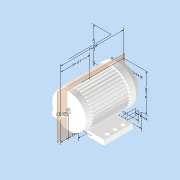
# Autodesk Inventor part: 43010400
Saved by Autodesk Inventor 2021 (Build 250183000, 183)
## iProperties
Category: PARTsolutions
Company: MAEDLER
Created: 2024-03-16
Part Number: 43010400
Material: Generic
Catalog Web Link: www.cadenas.de
Description: MAE-DNM-SM/I-B3-6/POLIG-Standard Three-Phase Motors SM/I, Model B3, 6-polig, approx. 1000 1/min.
Vendor: MAEDLER
Document SubType Name: Modeling
Designer: psAdmin
Manufacturer: MAEDLER
Mass: 6500 g
Surface Area: 2023.36 cm^2
Volume: 3410.98 cm^3
Density: 1 g/cm^3
Appearance: PSOLRGB-235-235-235
PSOL_IDENT_0: {$CADENAS_DATA/23d-libs/maedler/getriebe_u_getriebemotoren/drehstrom_normmotoren/d-nm_sm1_6pol_b3.pr
PSOL_IDENT_1: j},173 {VTYP=3D},{NB=43010400},{LINA=43010400},{NN=MAE-DNM-SM/I-B3-6/POLIG},{DATE=09.12.2023 00:31:4
PSOL_IDENT_2: 6},{GEOMDATE=01.12.2023 07:27:40},{VERSION=},{LINEID=20},{WBVAR=},{WBNUMERIC=}  {NB=43010400},{LINA=
PSOL_IDENT_3: 43010400},{KT=DUMMY},{ARTNR=43010400},{WEBSHOP=Produktdetails / Katalogseite / Montageanleitung},{MA
PSOL_IDENT_4: TK=Aluminium},{MAT=Rippengehäuse: Alu-Druckguss, Lagerschilder: Druckguss, Radiallüfter: Kunststoff,
PSOL_IDENT_5: Lüfterhaube: Stahlblech},{PDN=6-polig / ca. 1000 1/min.},{BG=71},{BF=B3},{IE=IE2},{LE=0.25},{DZ=900
PSOL_IDENT_6: },{J=0.0013},{LAN=59 / - / -},{STR=0.87},{LF=0.70},{NM=2.65},{ADM=2.1},{AS=4.0},{MDM=2.2},{GEW=6.5},
PSOL_IDENT_7: {CTN=85015100},{A=112},{B=90},{C=45},{D=14 j6},{E=30},{F=238},{G=185},{H=71},{K=7},{I=108},{L=137},{
PSOL_IDENT_8: P=24},{R=144},{S=10},{C1=85.5},{F1=280},{G1=125},{X=111},{Y=20},{W=88},{BK=5},{TK=16.0},{PGV=Pg11},{
PSOL_IDENT_9: GWB=M5 x 0.8},{DD=14},{FK=9.5},{XTK1=2.3},{GB1=5},{GB2=0.80},{Z=1},{KB=94},{KL=94},{IB=9.0},{KK=18.6
PSOL_IDENT_10: },{AL=24},{SW=22},{DIST=6.850}
NB: 43010400
NN: MAE-DNM-SM/I-B3-6/POLIG
NT: Standard Three-Phase Motors SM/I, Model B3, 6-polig, approx. 1000 1/min.
NBSYN: $ARTNR.
LINA: 43010400
CATALOG: Mädler
ARTNR: 43010400
WEBSHOP: https://maedler.de/ShopSearch?query=43010400
MATK: Aluminium
MAT: Finned housing: die-cast aluminium, end shields: Die-cast, radial fan: Plastic, fan cover: Sheet steel
PDN: 6 Poles / approx. 1000 1/min.
BG: 71
BF: B3
IE: IE2
LE: 0.25
DZ: 900
J: 0.0013
LAN: 59 / - / -
STR: 0.87
LF: 0.7
NM: 2.65
ADM: 2.1
AS: 4
MDM: 2.2
GEW: 6.5
CTN: 85015100
A: 112
B: 90
C: 45
D: 14 j6
E: 30
F: 238
G: 185
H: 71
K: 7
I: 108
L: 137
P: 24
R: 144
S: 10
G1: 125
X: 111
W: 88
BK: 5
TK: 16
PGV: Pg11
GWB: M5 x 0.8
SUPPLIER: MAEDLER
ARTICLENO: 43010400
BOMINFO: 43010400
CREATOR: CADENAS GmbH
Title: 43010400
Author: Cadenas PARTsolutions
Comments: Standard Three-Phase Motors SM/I, Model B3, 6-polig, approx. 1000 1/min.
Autodesk Inventor part; units mm, degrees
ref_plane "XZ Plane" through (0, 0, 0) normal (0, 1, 0) x (-1, 0, 0)
ref_plane "XY Plane" through (0, 0, 0) normal (0, 0, 1) x (1, 0, 0)
sketch "Skizze_3" plane through (0, 0, 0) normal (1, 0, 0) x (0, 1, 0)
  line L0 (0, 184) -> (0, 232)
  line L1 (7, 208) -> (10.5, 208)
  line L2 (10.5, 208) -> (10.5, 206)
  line L3 (10.5, 206) -> (63.9, 206)
  line L4 (63.9, 206) -> (63.9, 184)
  line L5 (63.9, 184) -> (0, 184)
  line L6 (0, 184) -> (0, 232)
  line L7 (7, 208) -> (7, 232)
  line L8 (7, 232) -> (0, 232)
  dimension "d64" = 2
  dimension "d65" = 3.5
  dimension "d68" = 53.4
  dimension "d69" = 22
  dimension "d70" = 63.9
  dimension "d71" = 24
  constraints: 18 end point, 1 perpendicular, 1 vertical
  measures "d64" distance of L1.end L2.end
  measures "d65" distance of L1.start L1.end
  measures "d68" distance of L2.end L3.end
  measures "d69" distance of L3.end L4.end
  measures "d70" distance of L4.end L5.end
  measures "d71" distance of L1.start L7.end
revolve "Revolution1" add sketch "Skizze_3" angle 360 about axis through (0, 0, 184) along (0, 0, -1)
sketch "Sketch_1" plane through (0, 0, 184) normal (0, 0, 1) x (1, 0, 0)
  arc A0 (-70.0009, 1.0346) -> (-70.0009, -1.0346) centre (-69.9647, 0) ccw
  line L0 (-70.0009, -1.0346) -> (-65.7533, -1.183)
  arc A1 (-63.8255, -3.0852) -> (-65.7533, -1.183) centre (-65.8231, -3.1818) ccw
  arc A2 (-63.8255, -3.0852) -> (-63.703, -5.0135) centre (0, 0) ccw
  arc A3 (-63.703, -5.0135) -> (-63.5223, -6.9373) centre (0, 0) ccw
  arc A4 (-65.1289, -9.1177) -> (-63.5223, -6.9373) centre (-65.5105, -7.1544) ccw
  line L1 (-65.1289, -9.1177) -> (-69.3009, -9.9286)
  arc A5 (-69.3009, -9.9286) -> (-68.9772, -11.9725) centre (-69.1033, -10.9449) ccw
  line L2 (-68.9772, -11.9725) -> (-64.7588, -11.4545)
  arc A6 (-62.5571, -13.0317) -> (-64.7588, -11.4545) centre (-64.515, -13.4396) ccw
  arc A7 (-62.5571, -13.0317) -> (-62.1344, -14.9172) centre (0, 0) ccw
  arc A8 (-62.1344, -14.9172) -> (-61.655, -16.789) centre (0, 0) ccw
  arc A9 (-62.9007, -19.1938) -> (-61.655, -16.789) centre (-63.5847, -17.3144) ccw
  line L3 (-62.9007, -19.1938) -> (-66.8945, -20.6474)
  arc A10 (-66.8945, -20.6474) -> (-66.255, -22.6155) centre (-66.5404, -21.6203) ccw
  line L4 (-66.255, -22.6155) -> (-62.1696, -21.444)
  arc A11 (-59.7483, -22.6573) -> (-62.1696, -21.444) centre (-61.6183, -23.3665) ccw
  arc A12 (-59.7483, -22.6573) -> (-59.0359, -24.4535) centre (0, 0) ccw
  arc A13 (-59.0359, -24.4535) -> (-58.2696, -26.2272) centre (0, 0) ccw
  arc A14 (-59.1237, -28.7974) -> (-58.2696, -26.2272) centre (-60.0933, -27.0481) ccw
  line L5 (-59.1237, -28.7974) -> (-62.8409, -30.8578)
  arc A15 (-62.8409, -30.8578) -> (-61.9015, -32.7016) centre (-62.339, -31.7633) ccw
  line L6 (-61.9015, -32.7016) -> (-58.0496, -30.9054)
  arc A16 (-55.4683, -31.7251) -> (-58.0496, -30.9054) centre (-57.2044, -32.718) ccw
  arc A17 (-55.4683, -31.7251) -> (-54.4837, -33.3877) centre (0, 0) ccw
  arc A18 (-54.4837, -33.3877) -> (-53.4493, -35.0197) centre (0, 0) ccw
  arc A19 (-53.8909, -37.6918) -> (-53.4493, -35.0197) centre (-55.1222, -36.1158) ccw
  line L7 (-53.8909, -37.6918) -> (-57.24, -40.3084)
  arc A20 (-57.24, -40.3084) -> (-56.0237, -41.9825) centre (-56.6027, -41.1242) ccw
  line L8 (-56.0237, -41.9825) -> (-52.5002, -39.6059)
  arc A21 (-49.8225, -40.0116) -> (-52.5002, -39.6059) centre (-51.3819, -41.264) ccw
  arc A22 (-49.8225, -40.0116) -> (-48.5899, -41.4997) centre (0, 0) ccw
  arc A23 (-48.5899, -41.4997) -> (-47.313, -42.9499) centre (0, 0) ccw
  arc A24 (-47.3311, -45.6582) -> (-47.313, -42.9499) centre (-48.7938, -44.2942) ccw
  line L9 (-47.3311, -45.6582) -> (-50.2297, -48.7665)
  arc A25 (-50.2297, -48.7665) -> (-48.7665, -50.2297) centre (-49.4725, -49.4725) ccw
  line L10 (-48.7665, -50.2297) -> (-45.6582, -47.3311)
  arc A26 (-42.9499, -47.313) -> (-45.6582, -47.3311) centre (-44.2942, -48.7938) ccw
  arc A27 (-42.9499, -47.313) -> (-41.4997, -48.5899) centre (0, 0) ccw
  arc A28 (-41.4997, -48.5899) -> (-40.0116, -49.8225) centre (0, 0) ccw
  arc A29 (-39.6059, -52.5002) -> (-40.0116, -49.8225) centre (-41.264, -51.3819) ccw
  line L11 (-39.6059, -52.5002) -> (-41.9825, -56.0237)
  arc A30 (-41.9825, -56.0237) -> (-40.3084, -57.24) centre (-41.1242, -56.6027) ccw
  line L12 (-40.3084, -57.24) -> (-37.6918, -53.8909)
  arc A31 (-35.0197, -53.4493) -> (-37.6918, -53.8909) centre (-36.1158, -55.1222) ccw
  arc A32 (-35.0197, -53.4493) -> (-33.3877, -54.4837) centre (0, 0) ccw
  arc A33 (-33.3877, -54.4837) -> (-31.7251, -55.4683) centre (0, 0) ccw
  arc A34 (-30.9054, -58.0496) -> (-31.7251, -55.4683) centre (-32.718, -57.2044) ccw
  line L13 (-30.9054, -58.0496) -> (-32.7016, -61.9015)
  arc A35 (-32.7016, -61.9015) -> (-30.8578, -62.8409) centre (-31.7633, -62.339) ccw
  line L14 (-30.8578, -62.8409) -> (-28.7974, -59.1237)
  arc A36 (-26.2272, -58.2696) -> (-28.7974, -59.1237) centre (-27.0481, -60.0933) ccw
  arc A37 (-26.2272, -58.2696) -> (-24.4535, -59.0359) centre (0, 0) ccw
  arc A38 (-24.4535, -59.0359) -> (-22.6573, -59.7483) centre (0, 0) ccw
  arc A39 (-21.444, -62.1696) -> (-22.6573, -59.7483) centre (-23.3665, -61.6183) ccw
  line L15 (-21.444, -62.1696) -> (-22.6155, -66.255)
  arc A40 (-22.6155, -66.255) -> (-20.6474, -66.8945) centre (-21.6203, -66.5404) ccw
  line L16 (-20.6474, -66.8945) -> (-19.1938, -62.9007)
  arc A41 (-16.789, -61.655) -> (-19.1938, -62.9007) centre (-17.3144, -63.5847) ccw
  arc A42 (-16.789, -61.655) -> (-14.9172, -62.1344) centre (0, 0) ccw
  arc A43 (-14.9172, -62.1344) -> (-13.0317, -62.5571) centre (0, 0) ccw
  arc A44 (-11.4545, -64.7588) -> (-13.0317, -62.5571) centre (-13.4396, -64.515) ccw
  line L17 (-11.4545, -64.7588) -> (-11.9725, -68.9772)
  arc A45 (-11.9725, -68.9772) -> (-9.9286, -69.3009) centre (-10.9449, -69.1033) ccw
  line L18 (-9.9286, -69.3009) -> (-9.1177, -65.1289)
  arc A46 (-6.9373, -63.5223) -> (-9.1177, -65.1289) centre (-7.1544, -65.5105) ccw
  arc A47 (-6.9373, -63.5223) -> (-5.0135, -63.703) centre (0, 0) ccw
  arc A48 (-5.0135, -63.703) -> (-3.0852, -63.8255) centre (0, 0) ccw
  arc A49 (-1.183, -65.7533) -> (-3.0852, -63.8255) centre (-3.1818, -65.8231) ccw
  line L19 (-1.183, -65.7533) -> (-1.0346, -70.0009)
  arc A50 (-1.0346, -70.0009) -> (1.0346, -70.0009) centre (0, -69.9647) ccw
  line L20 (1.0346, -70.0009) -> (1.183, -65.7533)
  arc A51 (3.0852, -63.8255) -> (1.183, -65.7533) centre (3.1818, -65.8231) ccw
  arc A52 (3.0852, -63.8255) -> (5.0135, -63.703) centre (0, 0) ccw
  arc A53 (5.0135, -63.703) -> (6.9373, -63.5223) centre (0, 0) ccw
  arc A54 (9.1177, -65.1289) -> (6.9373, -63.5223) centre (7.1544, -65.5105) ccw
  line L21 (9.1177, -65.1289) -> (9.9286, -69.3009)
  arc A55 (9.9286, -69.3009) -> (11.9725, -68.9772) centre (10.9449, -69.1033) ccw
  line L22 (11.9725, -68.9772) -> (11.4545, -64.7588)
  arc A56 (13.0317, -62.5571) -> (11.4545, -64.7588) centre (13.4396, -64.515) ccw
  arc A57 (13.0317, -62.5571) -> (14.9172, -62.1344) centre (0, 0) ccw
  arc A58 (14.9172, -62.1344) -> (16.789, -61.655) centre (0, 0) ccw
  arc A59 (19.1938, -62.9007) -> (16.789, -61.655) centre (17.3144, -63.5847) ccw
  line L23 (19.1938, -62.9007) -> (20.6474, -66.8945)
  arc A60 (20.6474, -66.8945) -> (22.6155, -66.255) centre (21.6203, -66.5404) ccw
  line L24 (22.6155, -66.255) -> (21.444, -62.1696)
  arc A61 (22.6573, -59.7483) -> (21.444, -62.1696) centre (23.3665, -61.6183) ccw
  arc A62 (22.6573, -59.7483) -> (24.4535, -59.0359) centre (0, 0) ccw
  arc A63 (24.4535, -59.0359) -> (26.2272, -58.2696) centre (0, 0) ccw
  arc A64 (28.7974, -59.1237) -> (26.2272, -58.2696) centre (27.0481, -60.0933) ccw
  line L25 (28.7974, -59.1237) -> (30.8578, -62.8409)
  arc A65 (30.8578, -62.8409) -> (32.7016, -61.9015) centre (31.7633, -62.339) ccw
  line L26 (32.7016, -61.9015) -> (30.9054, -58.0496)
  arc A66 (31.7251, -55.4683) -> (30.9054, -58.0496) centre (32.718, -57.2044) ccw
  arc A67 (31.7251, -55.4683) -> (33.3877, -54.4837) centre (0, 0) ccw
  arc A68 (33.3877, -54.4837) -> (35.0197, -53.4493) centre (0, 0) ccw
  arc A69 (37.6918, -53.8909) -> (35.0197, -53.4493) centre (36.1158, -55.1222) ccw
  line L27 (37.6918, -53.8909) -> (40.3084, -57.24)
  arc A70 (40.3084, -57.24) -> (41.9825, -56.0237) centre (41.1242, -56.6027) ccw
  line L28 (41.9825, -56.0237) -> (39.6059, -52.5002)
  arc A71 (40.0116, -49.8225) -> (39.6059, -52.5002) centre (41.264, -51.3819) ccw
  arc A72 (40.0116, -49.8225) -> (41.4997, -48.5899) centre (0, 0) ccw
  arc A73 (41.4997, -48.5899) -> (42.9499, -47.313) centre (0, 0) ccw
  arc A74 (45.6582, -47.3311) -> (42.9499, -47.313) centre (44.2942, -48.7938) ccw
  line L29 (45.6582, -47.3311) -> (48.7665, -50.2297)
  arc A75 (48.7665, -50.2297) -> (50.2297, -48.7665) centre (49.4725, -49.4725) ccw
  line L30 (50.2297, -48.7665) -> (47.3311, -45.6582)
  arc A76 (47.313, -42.9499) -> (47.3311, -45.6582) centre (48.7938, -44.2942) ccw
  arc A77 (47.313, -42.9499) -> (48.5899, -41.4997) centre (0, 0) ccw
  arc A78 (48.5899, -41.4997) -> (49.8225, -40.0116) centre (0, 0) ccw
  arc A79 (52.5002, -39.6059) -> (49.8225, -40.0116) centre (51.3819, -41.264) ccw
  line L31 (52.5002, -39.6059) -> (56.0237, -41.9825)
  arc A80 (56.0237, -41.9825) -> (57.24, -40.3084) centre (56.6027, -41.1242) ccw
  line L32 (57.24, -40.3084) -> (53.8909, -37.6918)
  arc A81 (53.4493, -35.0197) -> (53.8909, -37.6918) centre (55.1222, -36.1158) ccw
  arc A82 (53.4493, -35.0197) -> (54.4837, -33.3877) centre (0, 0) ccw
  arc A83 (54.4837, -33.3877) -> (55.4683, -31.7251) centre (0, 0) ccw
  arc A84 (58.0496, -30.9054) -> (55.4683, -31.7251) centre (57.2044, -32.718) ccw
  line L33 (58.0496, -30.9054) -> (61.9015, -32.7016)
  arc A85 (61.9015, -32.7016) -> (62.8409, -30.8578) centre (62.339, -31.7633) ccw
  line L34 (62.8409, -30.8578) -> (59.1237, -28.7974)
  arc A86 (58.2696, -26.2272) -> (59.1237, -28.7974) centre (60.0933, -27.0481) ccw
  arc A87 (58.2696, -26.2272) -> (59.0359, -24.4535) centre (0, 0) ccw
  arc A88 (59.0359, -24.4535) -> (59.7483, -22.6573) centre (0, 0) ccw
  arc A89 (62.1696, -21.444) -> (59.7483, -22.6573) centre (61.6183, -23.3665) ccw
  line L35 (62.1696, -21.444) -> (66.255, -22.6155)
  arc A90 (66.255, -22.6155) -> (66.8945, -20.6474) centre (66.5404, -21.6203) ccw
  line L36 (66.8945, -20.6474) -> (62.9007, -19.1938)
  arc A91 (61.655, -16.789) -> (62.9007, -19.1938) centre (63.5847, -17.3144) ccw
  arc A92 (61.655, -16.789) -> (62.1344, -14.9172) centre (0, 0) ccw
  arc A93 (62.1344, -14.9172) -> (62.5571, -13.0317) centre (0, 0) ccw
  arc A94 (64.7588, -11.4545) -> (62.5571, -13.0317) centre (64.515, -13.4396) ccw
  line L37 (64.7588, -11.4545) -> (68.9772, -11.9725)
  arc A95 (68.9772, -11.9725) -> (69.3009, -9.9286) centre (69.1033, -10.9449) ccw
  line L38 (69.3009, -9.9286) -> (65.1289, -9.1177)
  arc A96 (63.5223, -6.9373) -> (65.1289, -9.1177) centre (65.5105, -7.1544) ccw
  arc A97 (63.5223, -6.9373) -> (63.703, -5.0135) centre (0, 0) ccw
  arc A98 (63.703, -5.0135) -> (63.8255, -3.0852) centre (0, 0) ccw
  arc A99 (65.7533, -1.183) -> (63.8255, -3.0852) centre (65.8231, -3.1818) ccw
  line L39 (65.7533, -1.183) -> (70.0009, -1.0346)
  arc A100 (70.0009, -1.0346) -> (70.0009, 1.0346) centre (69.9647, 0) ccw
  line L40 (70.0009, 1.0346) -> (65.7533, 1.183)
  arc A101 (63.8255, 3.0852) -> (65.7533, 1.183) centre (65.8231, 3.1818) ccw
  arc A102 (63.8255, 3.0852) -> (63.703, 5.0135) centre (0, 0) ccw
  arc A103 (63.703, 5.0135) -> (63.5223, 6.9373) centre (0, 0) ccw
  arc A104 (65.1289, 9.1177) -> (63.5223, 6.9373) centre (65.5105, 7.1544) ccw
  line L41 (65.1289, 9.1177) -> (69.3009, 9.9286)
  arc A105 (69.3009, 9.9286) -> (68.9772, 11.9725) centre (69.1033, 10.9449) ccw
  line L42 (68.9772, 11.9725) -> (64.7588, 11.4545)
  arc A106 (62.5571, 13.0317) -> (64.7588, 11.4545) centre (64.515, 13.4396) ccw
  arc A107 (62.5571, 13.0317) -> (62.1344, 14.9172) centre (0, 0) ccw
  arc A108 (62.1344, 14.9172) -> (61.655, 16.789) centre (0, 0) ccw
  arc A109 (62.9007, 19.1938) -> (61.655, 16.789) centre (63.5847, 17.3144) ccw
  line L43 (62.9007, 19.1938) -> (66.8945, 20.6474)
  arc A110 (66.8945, 20.6474) -> (66.255, 22.6155) centre (66.5404, 21.6203) ccw
  line L44 (66.255, 22.6155) -> (62.1696, 21.444)
  arc A111 (59.7483, 22.6573) -> (62.1696, 21.444) centre (61.6183, 23.3665) ccw
  arc A112 (59.7483, 22.6573) -> (59.0359, 24.4535) centre (0, 0) ccw
  arc A113 (59.0359, 24.4535) -> (58.2696, 26.2272) centre (0, 0) ccw
  arc A114 (59.1237, 28.7974) -> (58.2696, 26.2272) centre (60.0933, 27.0481) ccw
  line L45 (59.1237, 28.7974) -> (62.8409, 30.8578)
  arc A115 (62.8409, 30.8578) -> (61.9015, 32.7016) centre (62.339, 31.7633) ccw
  line L46 (61.9015, 32.7016) -> (58.0496, 30.9054)
  arc A116 (55.4683, 31.7251) -> (58.0496, 30.9054) centre (57.2044, 32.718) ccw
  arc A117 (55.4683, 31.7251) -> (54.4837, 33.3877) centre (0, 0) ccw
  arc A118 (54.4837, 33.3877) -> (53.4493, 35.0197) centre (0, 0) ccw
  arc A119 (53.8909, 37.6918) -> (53.4493, 35.0197) centre (55.1222, 36.1158) ccw
  line L47 (53.8909, 37.6918) -> (57.24, 40.3084)
  arc A120 (57.24, 40.3084) -> (56.0237, 41.9825) centre (56.6027, 41.1242) ccw
  line L48 (56.0237, 41.9825) -> (52.5002, 39.6059)
  arc A121 (49.8225, 40.0116) -> (52.5002, 39.6059) centre (51.3819, 41.264) ccw
  arc A122 (49.8225, 40.0116) -> (48.5899, 41.4997) centre (0, 0) ccw
  arc A123 (48.5899, 41.4997) -> (47.313, 42.9499) centre (0, 0) ccw
  arc A124 (47.3311, 45.6582) -> (47.313, 42.9499) centre (48.7938, 44.2942) ccw
  line L49 (47.3311, 45.6582) -> (50.2297, 48.7665)
  arc A125 (50.2297, 48.7665) -> (48.7665, 50.2297) centre (49.4725, 49.4725) ccw
  line L50 (48.7665, 50.2297) -> (45.6582, 47.3311)
  arc A126 (42.9499, 47.313) -> (45.6582, 47.3311) centre (44.2942, 48.7938) ccw
  arc A127 (42.9499, 47.313) -> (41.4997, 48.5899) centre (0, 0) ccw
  arc A128 (41.4997, 48.5899) -> (40.0116, 49.8225) centre (0, 0) ccw
  arc A129 (39.6059, 52.5002) -> (40.0116, 49.8225) centre (41.264, 51.3819) ccw
  line L51 (39.6059, 52.5002) -> (41.9825, 56.0237)
  arc A130 (41.9825, 56.0237) -> (40.3084, 57.24) centre (41.1242, 56.6027) ccw
  line L52 (40.3084, 57.24) -> (37.6918, 53.8909)
  arc A131 (35.0197, 53.4493) -> (37.6918, 53.8909) centre (36.1158, 55.1222) ccw
  arc A132 (35.0197, 53.4493) -> (33.3877, 54.4837) centre (0, 0) ccw
  arc A133 (33.3877, 54.4837) -> (31.7251, 55.4683) centre (0, 0) ccw
  arc A134 (30.9054, 58.0496) -> (31.7251, 55.4683) centre (32.718, 57.2044) ccw
  line L53 (30.9054, 58.0496) -> (32.7016, 61.9015)
  arc A135 (32.7016, 61.9015) -> (30.8578, 62.8409) centre (31.7633, 62.339) ccw
  line L54 (30.8578, 62.8409) -> (28.7974, 59.1237)
  arc A136 (26.2272, 58.2696) -> (28.7974, 59.1237) centre (27.0481, 60.0933) ccw
  arc A137 (26.2272, 58.2696) -> (24.4535, 59.0359) centre (0, 0) ccw
  arc A138 (24.4535, 59.0359) -> (22.6573, 59.7483) centre (0, 0) ccw
  arc A139 (21.444, 62.1696) -> (22.6573, 59.7483) centre (23.3665, 61.6183) ccw
  line L55 (21.444, 62.1696) -> (22.6155, 66.255)
  arc A140 (22.6155, 66.255) -> (20.6474, 66.8945) centre (21.6203, 66.5404) ccw
  line L56 (20.6474, 66.8945) -> (19.1938, 62.9007)
  arc A141 (16.789, 61.655) -> (19.1938, 62.9007) centre (17.3144, 63.5847) ccw
  arc A142 (16.789, 61.655) -> (14.9172, 62.1344) centre (0, 0) ccw
  arc A143 (14.9172, 62.1344) -> (13.0317, 62.5571) centre (0, 0) ccw
  arc A144 (11.4545, 64.7588) -> (13.0317, 62.5571) centre (13.4396, 64.515) ccw
  line L57 (11.4545, 64.7588) -> (11.9725, 68.9772)
  arc A145 (11.9725, 68.9772) -> (9.9286, 69.3009) centre (10.9449, 69.1033) ccw
  line L58 (9.9286, 69.3009) -> (9.1177, 65.1289)
  arc A146 (6.9373, 63.5223) -> (9.1177, 65.1289) centre (7.1544, 65.5105) ccw
  arc A147 (6.9373, 63.5223) -> (5.0135, 63.703) centre (0, 0) ccw
  arc A148 (5.0135, 63.703) -> (3.0852, 63.8255) centre (0, 0) ccw
  arc A149 (1.183, 65.7533) -> (3.0852, 63.8255) centre (3.1818, 65.8231) ccw
  line L59 (1.183, 65.7533) -> (1.0346, 70.0009)
  arc A150 (1.0346, 70.0009) -> (-1.0346, 70.0009) centre (0, 69.9647) ccw
  line L60 (-1.0346, 70.0009) -> (-1.183, 65.7533)
  arc A151 (-3.0852, 63.8255) -> (-1.183, 65.7533) centre (-3.1818, 65.8231) ccw
  arc A152 (-3.0852, 63.8255) -> (-5.0135, 63.703) centre (0, 0) ccw
  arc A153 (-5.0135, 63.703) -> (-6.9373, 63.5223) centre (0, 0) ccw
  arc A154 (-9.1177, 65.1289) -> (-6.9373, 63.5223) centre (-7.1544, 65.5105) ccw
  line L61 (-9.1177, 65.1289) -> (-9.9286, 69.3009)
  arc A155 (-9.9286, 69.3009) -> (-11.9725, 68.9772) centre (-10.9449, 69.1033) ccw
  line L62 (-11.9725, 68.9772) -> (-11.4545, 64.7588)
  arc A156 (-13.0317, 62.5571) -> (-11.4545, 64.7588) centre (-13.4396, 64.515) ccw
  arc A157 (-13.0317, 62.5571) -> (-14.9172, 62.1344) centre (0, 0) ccw
  arc A158 (-14.9172, 62.1344) -> (-16.789, 61.655) centre (0, 0) ccw
  arc A159 (-19.1938, 62.9007) -> (-16.789, 61.655) centre (-17.3144, 63.5847) ccw
  line L63 (-19.1938, 62.9007) -> (-20.6474, 66.8945)
  arc A160 (-20.6474, 66.8945) -> (-22.6155, 66.255) centre (-21.6203, 66.5404) ccw
  line L64 (-22.6155, 66.255) -> (-21.444, 62.1696)
  arc A161 (-22.6573, 59.7483) -> (-21.444, 62.1696) centre (-23.3665, 61.6183) ccw
  arc A162 (-22.6573, 59.7483) -> (-24.4535, 59.0359) centre (0, 0) ccw
  arc A163 (-24.4535, 59.0359) -> (-26.2272, 58.2696) centre (0, 0) ccw
  arc A164 (-28.7974, 59.1237) -> (-26.2272, 58.2696) centre (-27.0481, 60.0933) ccw
  line L65 (-28.7974, 59.1237) -> (-30.8578, 62.8409)
  arc A165 (-30.8578, 62.8409) -> (-32.7016, 61.9015) centre (-31.7633, 62.339) ccw
  line L66 (-32.7016, 61.9015) -> (-30.9054, 58.0496)
  arc A166 (-31.7251, 55.4683) -> (-30.9054, 58.0496) centre (-32.718, 57.2044) ccw
  arc A167 (-31.7251, 55.4683) -> (-33.3877, 54.4837) centre (0, 0) ccw
  arc A168 (-33.3877, 54.4837) -> (-35.0197, 53.4493) centre (0, 0) ccw
  arc A169 (-37.6918, 53.8909) -> (-35.0197, 53.4493) centre (-36.1158, 55.1222) ccw
  line L67 (-37.6918, 53.8909) -> (-40.3084, 57.24)
  arc A170 (-40.3084, 57.24) -> (-41.9825, 56.0237) centre (-41.1242, 56.6027) ccw
  line L68 (-41.9825, 56.0237) -> (-39.6059, 52.5002)
  arc A171 (-40.0116, 49.8225) -> (-39.6059, 52.5002) centre (-41.264, 51.3819) ccw
  arc A172 (-40.0116, 49.8225) -> (-41.4997, 48.5899) centre (0, 0) ccw
  arc A173 (-41.4997, 48.5899) -> (-42.9499, 47.313) centre (0, 0) ccw
  arc A174 (-45.6582, 47.3311) -> (-42.9499, 47.313) centre (-44.2942, 48.7938) ccw
  line L69 (-45.6582, 47.3311) -> (-48.7665, 50.2297)
  arc A175 (-48.7665, 50.2297) -> (-50.2297, 48.7665) centre (-49.4725, 49.4725) ccw
  line L70 (-50.2297, 48.7665) -> (-47.3311, 45.6582)
  arc A176 (-47.313, 42.9499) -> (-47.3311, 45.6582) centre (-48.7938, 44.2942) ccw
  arc A177 (-47.313, 42.9499) -> (-48.5899, 41.4997) centre (0, 0) ccw
  arc A178 (-48.5899, 41.4997) -> (-49.8225, 40.0116) centre (0, 0) ccw
  arc A179 (-52.5002, 39.6059) -> (-49.8225, 40.0116) centre (-51.3819, 41.264) ccw
  line L71 (-52.5002, 39.6059) -> (-56.0237, 41.9825)
  arc A180 (-56.0237, 41.9825) -> (-57.24, 40.3084) centre (-56.6027, 41.1242) ccw
  line L72 (-57.24, 40.3084) -> (-53.8909, 37.6918)
  arc A181 (-53.4493, 35.0197) -> (-53.8909, 37.6918) centre (-55.1222, 36.1158) ccw
  arc A182 (-53.4493, 35.0197) -> (-54.4837, 33.3877) centre (0, 0) ccw
  arc A183 (-54.4837, 33.3877) -> (-55.4683, 31.7251) centre (0, 0) ccw
  arc A184 (-58.0496, 30.9054) -> (-55.4683, 31.7251) centre (-57.2044, 32.718) ccw
  line L73 (-58.0496, 30.9054) -> (-61.9015, 32.7016)
  arc A185 (-61.9015, 32.7016) -> (-62.8409, 30.8578) centre (-62.339, 31.7633) ccw
  line L74 (-62.8409, 30.8578) -> (-59.1237, 28.7974)
  arc A186 (-58.2696, 26.2272) -> (-59.1237, 28.7974) centre (-60.0933, 27.0481) ccw
  arc A187 (-58.2696, 26.2272) -> (-59.0359, 24.4535) centre (0, 0) ccw
  arc A188 (-59.0359, 24.4535) -> (-59.7483, 22.6573) centre (0, 0) ccw
  arc A189 (-62.1696, 21.444) -> (-59.7483, 22.6573) centre (-61.6183, 23.3665) ccw
  line L75 (-62.1696, 21.444) -> (-66.255, 22.6155)
  arc A190 (-66.255, 22.6155) -> (-66.8945, 20.6474) centre (-66.5404, 21.6203) ccw
  line L76 (-66.8945, 20.6474) -> (-62.9007, 19.1938)
  arc A191 (-61.655, 16.789) -> (-62.9007, 19.1938) centre (-63.5847, 17.3144) ccw
  arc A192 (-61.655, 16.789) -> (-62.1344, 14.9172) centre (0, 0) ccw
  arc A193 (-62.1344, 14.9172) -> (-62.5571, 13.0317) centre (0, 0) ccw
  arc A194 (-64.7588, 11.4545) -> (-62.5571, 13.0317) centre (-64.515, 13.4396) ccw
  line L77 (-64.7588, 11.4545) -> (-68.9772, 11.9725)
  arc A195 (-68.9772, 11.9725) -> (-69.3009, 9.9286) centre (-69.1033, 10.9449) ccw
  line L78 (-69.3009, 9.9286) -> (-65.1289, 9.1177)
  arc A196 (-63.5223, 6.9373) -> (-65.1289, 9.1177) centre (-65.5105, 7.1544) ccw
  arc A197 (-63.5223, 6.9373) -> (-63.703, 5.0135) centre (0, 0) ccw
  arc A198 (-63.703, 5.0135) -> (-63.8255, 3.0852) centre (0, 0) ccw
  arc A199 (-65.7533, 1.183) -> (-63.8255, 3.0852) centre (-65.8231, 3.1818) ccw
  line L79 (-65.7533, 1.183) -> (-70.0009, 1.0346)
  constraints: 400 point on circle, 200 centre point, 160 end point
extrude "Extrusion1" add sketch "Sketch_1" against normal blind 138
sketch "Sketch_2" plane through (0, 0, 0) normal (1, 0, 0) x (0, 0, -1)
  line L0 (0, 0) -> (-46, 0)
  line L1 (-46, 0) -> (-46, 71)
  line L2 (-46, 71) -> (-23.3906, 71)
  line L3 (-23.3906, 71) -> (0, 57.4954)
  line L4 (0, 57.4954) -> (0, 0)
  line L5 (0, 0) -> (-46, 0)
  constraints: 12 end point
revolve "Revolution2" add sketch "Sketch_2" angle 360 about axis through (0, 0, 0) along (0, 0, -1)
sketch "Sketch_7" plane through (0, 0, 184) normal (0, 0, 1) x (1, 0, 0)
  arc A0 (-36.5, -63.2199) -> (36.5, -63.2199) centre (0, 0) ccw
  line L0 (36.5, -63.2199) -> (31.95, -55.339)
  arc A1 (-31.95, -55.339) -> (31.95, -55.339) centre (0, 0) ccw
  line L1 (-31.95, -55.339) -> (-36.5, -63.2199)
  constraints: 4 end point, 4 point on circle, 2 centre point
extrude "Extrusion5" cut sketch "Sketch_7" against normal blind 138
sketch "Sketch_11" plane through (0, 0, 172) normal (0, 0, 1) x (1, 0, 0)
  line L0 (22.3194, -61.4468) -> (40.8726, -80)
  line L1 (98.5, -61) -> (44.5, -61)
  line L2 (44.5, -61) -> (34.8974, -51.3974)
  arc A0 (22.3194, -61.4468) -> (34.8974, -51.3974) centre (-9.8435, -8.2955) ccw
  line L3 (98.5, -80) -> (40.8726, -80)
  line L4 (98.5, -61) -> (98.5, -80)
  circle A1 centre (0, 0) radius 7 projected
  line L5 (0, 0) -> (0, -120.8726)
  line L6 (-22.3194, -61.4468) -> (-40.8726, -80)
  line L7 (-98.5, -61) -> (-44.5, -61)
  line L8 (-44.5, -61) -> (-34.8974, -51.3974)
  arc A2 (-34.8974, -51.3974) -> (-22.3194, -61.4468) centre (9.8435, -8.2955) ccw
  line L9 (-98.5, -80) -> (-40.8726, -80)
  line L10 (-98.5, -61) -> (-98.5, -80)
  dimension "d55" = 16
  constraints: 22 end point, 7 symmetric about line, 4 point on circle, 2 centre point, 1 vertical, 2 other
  measures "d55" distance between parallel lines of L2 L0
extrude "Extrusion6" add sketch "Sketch_11" against normal blind 108 contours A0 L2 L1 L4 L3 L0 | L6 L9 L10 L7 L8 A2
sketch "Sketch19" plane through (44.5, -61, 172) normal (0, 1, 0) x (1, 0, 0)
  line L0 (54, 0) -> (0, 0) projected
  line L1 (54, 0) -> (26.5, 0)
  line L2 (26.5, -12) -> (26.5, 126) projected
  line L3 (54, 108) -> (-3.6274, 108) projected
  line L4 (40.25, 54) -> (40.25, 24)
  line L5 (54, 54) -> (26.5, 54)
  line L6 (54, 0) -> (54, 108) projected
  line L7 (54, 24) -> (26.5, 24)
  circle A0 centre (40.25, 54) radius 7
  circle A1 centre (40.25, 24) radius 7
  circle A2 centre (40.25, 84) radius 7
  point P0 (-44.5, 172)
  dimension "d57" = 14
  dimension "d58" = 14
  dimension "d61" = 30
  constraints: 8 end point, 4 point on line, 3 centre point, 3 midpoint, 2 horizontal, 1 coincident, 1 perpendicular, 1 symmetric about line, 2 other
  measures "d57" diameter of A0
  measures "d58" diameter of A1
  measures "d61" distance of L4.start L4.end
extrude "Extrusion9" cut sketch "Sketch19" against normal through all contours A1 L7 | L7 L4 A1 | A1 L4 L7 | A0 L4 L5 | L5 A0 | L5 L4 A0 | A2
mirror "Mirror1" about plane through (0, 0, 0) normal (1, 0, 0) of "Extrusion9"
chamfer "Chamfer1" distance 1 angle 45 1 edges at (0, -7, 232)
ref_plane "Work Plane1" through (-7, 0, 0) normal (1, 0, 0) x (0, 1, 0)
sketch "Sketch20" plane through (-7, 0, 0) normal (1, 0, 0) x (0, 1, 0)
  line L0 (-6, 232) -> (6, 232) projected
  line L1 (-10.5, 208) -> (10.5, 208) projected
  arc A0 (-2, 214.975) -> (2, 214.975) centre (0, 214.975) ccw
  arc A1 (2, 222.975) -> (-2, 222.975) centre (0, 222.975) ccw
  line L2 (2, 214.975) -> (2, 222.975)
  line L3 (-2, 222.975) -> (-2, 214.975)
  point P0 (0, 0)
  point P1 (0, 224.975)
  dimension "d81" = 2
  dimension "d82" = 2
  constraints: 5 point on circle, 4 end point, 2 centre point, 2 vertical, 1 other
  measures "d81" radius of A1
  measures "d82" radius of A0
extrude "Extrusion10" cut sketch "Sketch20" along normal blind 3
chamfer "Chamfer2" distance 0.25 angle 45 6 edges at (-6.7082, 2, 218.975) (-6.8338, 1.5165, 224.279) (-6.8555, -1.4149, 224.3885) (-6.7082, -2, 218.975) (-6.8349, -1.5111, 213.6648) (-6.8415, 1.481, 213.6309)
fillet "Fillet1" radius 0.25 4 edges at (-4, 0, 212.975) (-4, 2, 218.975) (-4, 0, 224.975) (-4, -2, 218.975)
body "Solid1"
